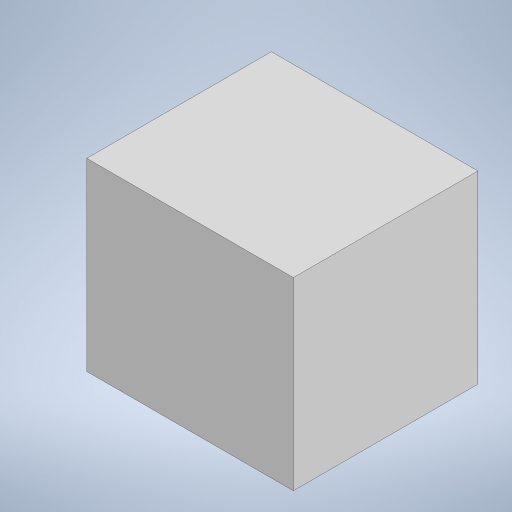
# Autodesk Inventor part: NEMA 17 Completely Correct
Saved by Autodesk Inventor 2024 (Build 280153000, 153)
## iProperties
Created: 2025-02-04
Part Number: NEMA 17 Completely Correct
Material: Generic
Document SubType Name: Modeling
Designer: Sven
Density: 1 g/cm^3
Appearance: Default
Author: Sven
Autodesk Inventor part; units mm, degrees
ref_plane "YZ Plane" through (0, 0, 0) normal (1, 0, 0) x (0, 1, 0)
ref_plane "XZ Plane" through (0, 0, 0) normal (0, 1, 0) x (-1, 0, 0)
ref_plane "XY Plane" through (0, 0, 0) normal (0, 0, 1) x (1, 0, 0)
sketch "Sketch1" plane through (0, 0, 0) normal (1, 0, 0) x (0, 1, 0)
  line L0 (21, 21) -> (-21, 21)
  line L1 (-21, 21) -> (-21, -21)
  line L2 (-21, -21) -> (21, -21)
  line L3 (21, -21) -> (21, 21)
  point P0 (0, 0)
  point P1 (0, 21)
  point P2 (21, 0)
  dimension "d0" = 42
  dimension "d1" = 42
  constraints: 8 end point, 2 midpoint, 2 parallel, 1 horizontal, 1 horizontal alignment, 1 perpendicular, 1 vertical alignment
  measures "d0" distance of L2.end L0.start
  measures "d1" distance of L1.end L2.end
extrude "Extrusion1" add sketch "Sketch1" along normal blind 47
sketch "Sketch2" plane through (0, 0, 0) normal (-1, 0, 0) x (0, 0, 1)
  circle A0 centre (0, 0) radius 2.5
  dimension "d4" = 5
  constraints: 1 centre point, 1 coincident
  measures "d4" diameter of A0
extrude "Extrusion2" add sketch "Sketch2" along normal blind 12
sketch "Sketch3" plane through (0, 0, 0) normal (-1, 0, 0) x (0, 0, 1)
  circle A0 centre (15.5, 15.5) radius 2
  line L0 (-13.7584, 0) -> (4.183, 0) construction
  line L1 (0, 11.541) -> (0, -2.5) construction
  circle A1 centre (0, 0) radius 2.5 construction
  circle A2 centre (15.5, -15.5) radius 2
  circle A3 centre (-15.5, 15.5) radius 2
  circle A4 centre (-15.5, -15.5) radius 2
  dimension "d7" = 15.5
  dimension "d8" = 15.5
  dimension "d9" = 4
  constraints: 4 centre point, 4 end point, 3 symmetric about line, 1 horizontal, 1 vertical, 1 vertical alignment, 4 other
  measures "d7" horizontal distance of point (0, 0) A0.centre
  measures "d8" horizontal distance of point (0, 0) A0.centre
  measures "d9" diameter of A0
extrude "Extrusion3" cut sketch "Sketch3" against normal blind 12
body "Solid1"
